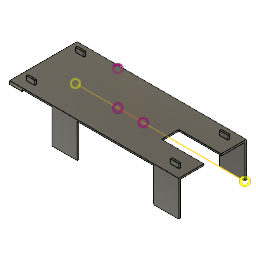
support v17 (Autodesk Fusion 360 design; units mm, degrees)
Autodesk Fusion 360 part; units mm, degrees
sketch "Sketch1" plane through (0, 0, 0) normal (0, 0, 1) x (1, 0, 0)
  line L0 (0, 0) -> (200, 0)
  line L1 (200, 0) -> (200, 80)
  line L2 (200, 80) -> (0, 80)
  line L3 (0, 80) -> (0, 0)
  dimension "d1" = 200
  dimension "d2" = 80
  dimension "d58" = 0
  dimension "d59" = 0
  dimension "d60" = 0
  dimension "d61" = 0
  dimension "d125" = 0
  dimension "d126" = 0
  dimension "d127" = 0
  dimension "d128" = 0
extrude "Extrude1" add sketch "Sketch1" along normal blind 2
sketch "Sketch2" plane through (0, 0, 2) normal (0, 0, 1) x (-1, 0, 0)
  line L0 (0, -80) -> (0, 0)
  line L1 (0, 0) -> (-200, 0)
  line L2 (-200, 0) -> (-200, -80)
  line L3 (-200, -80) -> (0, -80)
  line L4 (-10, -70) -> (-20, -70)
  line L5 (-20, -70) -> (-20, -68)
  line L6 (-20, -68) -> (-10, -68)
  line L7 (-10, -68) -> (-10, -70)
  dimension "d5" = 10
  dimension "d6" = 2
  dimension "d9" = 10
  dimension "d10" = 10
  measures "d5" distance of L0.end
  measures "d9" distance of L3 L4
  measures "d10" distance of L0 L7
extrude "Extrude2" add sketch "Sketch2" along normal blind 5 contours L4 L5 L6 L7
sketch "Sketch3" plane through (0, 0, 2) normal (0, 0, 1) x (-1, 0, 0)
  line L0 (-10, -68) -> (-10, -70)
  line L1 (-10, -70) -> (-20, -70)
  line L2 (-20, -70) -> (-20, -68)
  line L3 (-20, -68) -> (-10, -68)
  line L4 (0, -80) -> (0, 0)
  line L5 (0, 0) -> (-200, 0)
  line L6 (-200, 0) -> (-200, -80)
  line L7 (-200, -80) -> (0, -80)
  line L8 (-10, -10) -> (-20, -10)
  line L9 (-20, -10) -> (-20, -12)
  line L10 (-20, -12) -> (-10, -12)
  line L11 (-10, -12) -> (-10, -10)
  dimension "d11" = 10
  dimension "d12" = 2
  dimension "d13" = 10
  dimension "d14" = 10
  measures "d13" distance of L5 L8
  measures "d14" distance of L4 L11
extrude "Extrude3" add sketch "Sketch3" along normal blind 5 contours L8 L9 L10 L11
sketch "Sketch4" plane through (0, 0, 2) normal (0, 0, 1) x (-1, 0, 0)
  line L0 (-10, -12) -> (-20, -12)
  line L1 (-20, -12) -> (-20, -10)
  line L2 (-20, -10) -> (-10, -10)
  line L3 (-10, -10) -> (-10, -12)
  line L4 (-10, -68) -> (-10, -70)
  line L5 (-10, -70) -> (-20, -70)
  line L6 (-20, -70) -> (-20, -68)
  line L7 (-20, -68) -> (-10, -68)
  line L8 (0, -80) -> (0, 0)
  line L9 (0, 0) -> (-200, 0)
  line L10 (-200, 0) -> (-200, -80)
  line L11 (-200, -80) -> (0, -80)
  line L12 (-190, -10) -> (-180, -10)
  line L13 (-180, -10) -> (-180, -12)
  line L14 (-180, -12) -> (-190, -12)
  line L15 (-190, -12) -> (-190, -10)
  dimension "d17" = 10
  dimension "d18" = 2
  dimension "d19" = 10
  dimension "d20" = 10
  measures "d20" distance of L9 L12
extrude "Extrude4" add sketch "Sketch4" along normal blind 5 contours L12 L13 L14 L15
sketch "Sketch5" plane through (0, 0, 2) normal (0, 0, 1) x (-1, 0, 0)
  line L0 (-190, -12) -> (-190, -10)
  line L1 (-190, -10) -> (-180, -10)
  line L2 (-180, -10) -> (-180, -12)
  line L3 (-180, -12) -> (-190, -12)
  line L4 (-10, -12) -> (-20, -12)
  line L5 (-20, -12) -> (-20, -10)
  line L6 (-20, -10) -> (-10, -10)
  line L7 (-10, -10) -> (-10, -12)
  line L8 (-10, -68) -> (-10, -70)
  line L9 (-10, -70) -> (-20, -70)
  line L10 (-20, -70) -> (-20, -68)
  line L11 (-20, -68) -> (-10, -68)
  line L12 (0, -80) -> (0, 0)
  line L13 (0, 0) -> (-200, 0)
  line L14 (-200, 0) -> (-200, -80)
  line L15 (-200, -80) -> (0, -80)
  line L16 (-190, -70) -> (-180, -70)
  line L17 (-180, -70) -> (-180, -68)
  line L18 (-180, -68) -> (-190, -68)
  line L19 (-190, -68) -> (-190, -70)
  dimension "d23" = 10
  dimension "d24" = 2
  dimension "d25" = 10
  dimension "d26" = 10
  measures "d25" distance of L14 L19
  measures "d26" distance of L15 L16
extrude "Extrude5" add sketch "Sketch5" along normal blind 5 contours L16 L17 L18 L19
sketch "Sketch8" plane through (0, 0, 0) normal (0, 0, 1) x (1, 0, 0)
  line L0 (20.5, 3) -> (120.5, 3)
  line L1 (120.5, 3) -> (120.5, 4)
  line L2 (120.5, 4) -> (20.5, 4)
  line L3 (20.5, 4) -> (20.5, 3)
  line L4 (0, 0) -> (200, 0)
  line L5 (0, 80) -> (0, 0)
  dimension "d42" = 100
  dimension "d43" = 1
  dimension "d44" = 3
  dimension "d45" = 20.5
  measures "d44" distance of L0 L4
  measures "d45" distance of L3 L5
extrude "Extrude8" add sketch "Sketch8" against normal blind 3
sketch "Sketch9" plane through (0, 0, 0) normal (0, 0, -1) x (1, 0, 0)
  line L0 (20.5, -3) -> (120.5, -3)
  line L1 (120.5, -3) -> (120.5, -4)
  line L2 (120.5, -4) -> (20.5, -4)
  line L3 (20.5, -4) -> (20.5, -3)
  line L4 (0, 0) -> (0, -80)
  line L5 (0, -80) -> (200, -80)
  line L6 (200, -80) -> (200, 0)
  line L7 (200, 0) -> (0, 0)
  line L8 (20.5, -77) -> (120.5, -77)
  line L9 (120.5, -77) -> (120.5, -76)
  line L10 (120.5, -76) -> (20.5, -76)
  line L11 (20.5, -76) -> (20.5, -77)
  dimension "d48" = 100
  dimension "d49" = 1
  dimension "d50" = 3
  dimension "d51" = 20.5
  measures "d50" distance of L5 L8
  measures "d51" distance of L4 L11
extrude "Extrude9" add sketch "Sketch9" along normal blind 3 contours L8 L9 L10 L11
sketch "Sketch10" plane through (0, 0, 0) normal (0, 0, -1) x (1, 0, 0)
  line L0 (20.5, -76) -> (120.5, -76)
  line L1 (120.5, -76) -> (120.5, -77)
  line L2 (120.5, -77) -> (20.5, -77)
  line L3 (20.5, -77) -> (20.5, -76)
  line L4 (20.5, -3) -> (120.5, -3)
  line L5 (120.5, -3) -> (120.5, -4)
  line L6 (120.5, -4) -> (20.5, -4)
  line L7 (20.5, -4) -> (20.5, -3)
  line L8 (0, 0) -> (0, -80)
  line L9 (0, -80) -> (200, -80)
  line L10 (200, -80) -> (200, 0)
  line L11 (200, 0) -> (0, 0)
  line L12 (200, -80) -> (170, -80)
  line L13 (170, -80) -> (170, -78)
  line L14 (170, -78) -> (200, -78)
  line L15 (200, -78) -> (200, -80)
  dimension "d66" = 30
  dimension "d67" = 2
extrude "Extrude10" add sketch "Sketch10" along normal blind 40 contours L9 L10 L12 L13 L14 L15
sketch "Sketch11" plane through (0, 0, 0) normal (0, 0, -1) x (1, 0, 0)
  line L0 (170, -80) -> (170, -78)
  line L1 (170, -78) -> (200, -78)
  line L2 (200, -78) -> (200, 0)
  line L3 (200, 0) -> (0, 0)
  line L4 (0, 0) -> (0, -80)
  line L5 (0, -80) -> (170, -80)
  line L6 (20.5, -3) -> (120.5, -3)
  line L7 (120.5, -3) -> (120.5, -4)
  line L8 (120.5, -4) -> (20.5, -4)
  line L9 (20.5, -4) -> (20.5, -3)
  line L10 (20.5, -76) -> (120.5, -76)
  line L11 (120.5, -76) -> (120.5, -77)
  line L12 (120.5, -77) -> (20.5, -77)
  line L13 (20.5, -77) -> (20.5, -76)
  line L14 (200, 0) -> (170, 0)
  line L15 (170, 0) -> (170, -2)
  line L16 (170, -2) -> (200, -2)
  line L17 (200, -2) -> (200, 0)
  dimension "d70" = 2
  dimension "d71" = 30
  measures "d70" distance of L3.end
extrude "Extrude11" add sketch "Sketch11" along normal blind 40 contours L2 L3 L14 L15 L16 L17
sketch "Sketch12" plane through (0, 0, 0) normal (0, 0, -1) x (1, 0, 0)
  line L0 (170, -2) -> (170, 0)
  line L1 (170, 0) -> (0, 0)
  line L2 (0, 0) -> (0, -80)
  line L3 (0, -80) -> (170, -80)
  line L4 (170, -80) -> (170, -78)
  line L5 (170, -78) -> (200, -78)
  line L6 (200, -78) -> (200, -2)
  line L7 (200, -2) -> (170, -2)
  line L8 (20.5, -3) -> (120.5, -3)
  line L9 (120.5, -3) -> (120.5, -4)
  line L10 (120.5, -4) -> (20.5, -4)
  line L11 (20.5, -4) -> (20.5, -3)
  line L12 (20.5, -76) -> (120.5, -76)
  line L13 (120.5, -76) -> (120.5, -77)
  line L14 (120.5, -77) -> (20.5, -77)
  line L15 (20.5, -77) -> (20.5, -76)
  line L16 (50, 0) -> (80, 0)
  line L17 (80, 0) -> (80, -2)
  line L18 (80, -2) -> (50, -2)
  line L19 (50, -2) -> (50, 0)
  dimension "d74" = 30
  dimension "d75" = 2
  dimension "d78" = 50
  measures "d75" distance of L1.end
  measures "d78" distance of L2 L19
extrude "Extrude12" add sketch "Sketch12" along normal blind 40 contours L1 L16 L17 L18 L19
sketch "Sketch13" plane through (0, 0, 0) normal (0, 0, -1) x (1, 0, 0)
  line L0 (20.5, -76) -> (120.5, -76)
  line L1 (120.5, -76) -> (120.5, -77)
  line L2 (120.5, -77) -> (20.5, -77)
  line L3 (20.5, -77) -> (20.5, -76)
  line L4 (20.5, -3) -> (120.5, -3)
  line L5 (120.5, -3) -> (120.5, -4)
  line L6 (120.5, -4) -> (20.5, -4)
  line L7 (20.5, -4) -> (20.5, -3)
  line L8 (80, 0) -> (80, -2)
  line L9 (80, -2) -> (50, -2)
  line L10 (50, -2) -> (50, 0)
  line L11 (50, 0) -> (0, 0)
  line L12 (0, 0) -> (0, -80)
  line L13 (0, -80) -> (170, -80)
  line L14 (170, -80) -> (170, -78)
  line L15 (170, -78) -> (200, -78)
  line L16 (200, -78) -> (200, -2)
  line L17 (200, -2) -> (170, -2)
  line L18 (170, -2) -> (170, 0)
  line L19 (170, 0) -> (80, 0)
  line L20 (50, -80) -> (80, -80)
  line L21 (80, -80) -> (80, -78)
  line L22 (80, -78) -> (50, -78)
  line L23 (50, -78) -> (50, -80)
  dimension "d79" = 30
  dimension "d80" = 2
  dimension "d81" = 50
  dimension "d175" = 76
  measures "d81" distance of L12 L23
  measures "d175" distance of L11.end
extrude "Extrude13" add sketch "Sketch13" along normal blind 40 contours L13 L20 L21 L22 L23
sketch "Sketch17" plane through (200, 0, 0) normal (1, 0, 0) x (0, 1, 0)
  line L0 (2, 0) -> (78, 0)
  line L1 (78, 0) -> (78, -40)
  line L2 (78, -40) -> (80, -40)
  line L3 (80, -40) -> (80, 2)
  line L4 (80, 2) -> (0, 2)
  line L5 (0, 2) -> (0, -40)
  line L6 (0, -40) -> (2, -40)
  line L7 (2, -40) -> (2, 0)
  line L8 (30, 2) -> (50, 2)
  line L9 (50, 2) -> (50, 0)
  line L10 (50, 0) -> (30, 0)
  line L11 (30, 0) -> (30, 2)
  dimension "d115" = 20
  dimension "d116" = 2
  dimension "d117" = 30
  dimension "d118" = 28.4712
  measures "d116" distance of origin
  measures "d117" distance of L5
  measures "d118" distance of L3 L9
extrude "Extrude15" cut sketch "Sketch17" against normal blind 50 contours L0 L4 L8 L9 L10 L11
sketch "Sketch21" plane through (0, 0, 0) normal (0, 0, -1) x (1, 0, 0)
  line L0 (20.5, -3) -> (120.5, -3)
  line L1 (120.5, -3) -> (120.5, -4)
  line L2 (120.5, -4) -> (20.5, -4)
  line L3 (20.5, -4) -> (20.5, -3)
  line L4 (20.5, -76) -> (120.5, -76)
  line L5 (120.5, -76) -> (120.5, -77)
  line L6 (120.5, -77) -> (20.5, -77)
  line L7 (20.5, -77) -> (20.5, -76)
  line L8 (200, -50) -> (150, -50)
  line L9 (150, -50) -> (150, -30)
  line L10 (150, -30) -> (200, -30)
  line L11 (200, -30) -> (200, -2)
  line L12 (200, -2) -> (170, -2)
  line L13 (170, -2) -> (170, 0)
  line L14 (170, 0) -> (80, 0)
  line L15 (80, 0) -> (80, -2)
  line L16 (80, -2) -> (50, -2)
  line L17 (50, -2) -> (50, 0)
  line L18 (50, 0) -> (0, 0)
  line L19 (0, 0) -> (0, -80)
  line L20 (0, -80) -> (50, -80)
  line L21 (50, -80) -> (50, -78)
  line L22 (50, -78) -> (80, -78)
  line L23 (80, -78) -> (80, -80)
  line L24 (80, -80) -> (170, -80)
  line L25 (170, -80) -> (170, -78)
  line L26 (170, -78) -> (200, -78)
  line L27 (200, -78) -> (200, -50)
  line L28 (0, -80) -> (15, -80)
  line L29 (15, -80) -> (15, 0)
  line L30 (15, 0) -> (0, 0)
  line L31 (0, 0) -> (0, -80)
extrude "Extrude20" add sketch "Sketch21" along normal blind 2 contours L18 L19 L20 L28 L29 L30 L31
sketch "Sketch23" plane through (0, 0, -2) normal (0, 0, -1) x (1, 0, 0)
  line L0 (0, 0) -> (0, -80)
  line L1 (0, -80) -> (15, -80)
  line L2 (15, -80) -> (15, 0)
  line L3 (15, 0) -> (0, 0)
  line L4 (15, -40) -> (0, -40)
  line L5 (0, -40) -> (0, -48)
  line L6 (0, -48) -> (15, -48)
  line L7 (15, -48) -> (15, -40)
  dimension "d168" = 8
extrude "Extrude21" add sketch "Sketch23" along normal blind 1 contours L0 L2 L4 L5 L6 L7
sketch "Sketch24" plane through (0, 78, 0) normal (0, -1, 0) x (1, 0, 0)
  line L0 (80, 0) -> (50, 0)
  line L1 (50, 0) -> (50, -40)
  line L2 (50, -40) -> (80, -40)
  line L3 (80, -40) -> (80, 0)
  line L4 (80, -40) -> (50, -40)
  line L5 (0, -40) -> (200, -40)
  line L6 (50, -40) -> (80, -40)
  dimension "d171" = 0
  dimension "d172" = 0
  dimension "d173" = 0
  dimension "d174" = 40
  measures "d171" distance of L4 L5
  measures "d172" distance of L4 L5
  measures "d173" distance of L4 L5
